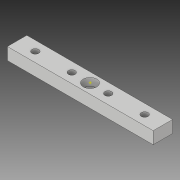
# Autodesk Inventor part: flowmeter_mount
Saved by Autodesk Inventor 2019 (Build 230136000, 136)
## iProperties
Created: 2019-12-12
Part Number: flowmeter_mount
Material: Generic
Document SubType Name: Modeling
Designer: devon
Density: 1 g/cm^3
Appearance: Default
Author: devon
Autodesk Inventor part; units mm, degrees
ref_plane "YZ Plane" through (0, 0, 0) normal (1, 0, 0) x (0, 1, 0)
ref_plane "XZ Plane" through (0, 0, 0) normal (0, 1, 0) x (-1, 0, 0)
ref_plane "XY Plane" through (0, 0, 0) normal (0, 0, 1) x (1, 0, 0)
sketch "Sketch1" plane through (0, 0, 0) normal (0, 1, 0) x (-1, 0, 0)
  line L0 (60, 8) -> (-60, 8)
  line L1 (-60, 8) -> (-60, -8)
  line L2 (-60, -8) -> (60, -8)
  line L3 (60, -8) -> (60, 8)
  line L4 (60, 8) -> (-60, -8) construction
  line L5 (-60, 8) -> (60, -8) construction
  point P0 (0, 0)
  dimension "d0" = 16
  dimension "d1" = 120
  constraints: 12 end point, 2 midpoint, 2 parallel, 1 horizontal, 1 perpendicular
  measures "d0" distance of L2.end L0.start
  measures "d1" distance of L1.end L2.end
extrude "Extrusion1" add sketch "Sketch1" along normal blind 10
hole "Hole1" at (0, 10, 0) direction (0, -1, 0) diameter 7.142 depth 25.4 counterbore diameter 11.113 counterbore depth 6.35 clearance for "Socket Head Cap Screw" size "1/4" standard "Ansi Unified Screw Threads"
sketch "Sketch2" plane through (0, 10, 0) normal (0, 1, 0) x (1, 0, 0)
  circle A0 centre (15, 0) radius 2.75
  circle A1 centre (45, 0) radius 2.75
  circle A2 centre (-15, 0) radius 2.75
  circle A3 centre (-45, 0) radius 2.75
  point P0 (0, 0)
  dimension "d15" = 5.5
  dimension "d16" = 15
  dimension "d17" = 30
  dimension "d18" = 5.5
  dimension "d19" = 15
  dimension "d20" = 5.5
  dimension "d21" = 30
  dimension "d22" = 5.5
  constraints: 4 centre point
  measures "d15" diameter of A0
  measures "d16" distance of point (0, 0) A0.centre
  measures "d17" distance of A0.centre A1.centre
  measures "d18" diameter of A1
  measures "d19" distance of point (0, 0) A2.centre
  measures "d20" diameter of A2
  measures "d21" distance of A2.centre A3.centre
  measures "d22" diameter of A3
extrude "Extrusion2" cut sketch "Sketch2" against normal up to next
body "Solid1"
